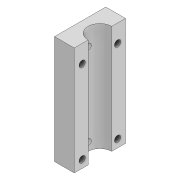
# Autodesk Inventor part: Tube_outerhole_template_p2
Saved by Autodesk Inventor 2022 (Build 260153000, 153)
## iProperties
Created: 2022-05-02
Part Number: Tube_outerhole_template_p2
Material: Generic
Document SubType Name: Modeling
Designer: dell
Density: 1 g/cm^3
Appearance: Default
Author: dell
Autodesk Inventor part; units mm, degrees
ref_plane "YZ Plane" through (0, 0, 0) normal (1, 0, 0) x (0, 1, 0)
ref_plane "XZ Plane" through (0, 0, 0) normal (0, 1, 0) x (-1, 0, 0)
ref_plane "XY Plane" through (0, 0, 0) normal (0, 0, 1) x (1, 0, 0)
sketch "Sketch1" plane through (0, 0, 0) normal (0, 1, 0) x (-1, 0, 0)
  circle A0 centre (0, 0) radius 6
  line L0 (10, 13) -> (-10, 13)
  line L1 (-10, 13) -> (-10, -13)
  line L2 (-10, -13) -> (10, -13)
  line L3 (10, -13) -> (10, 13)
  dimension "d0" = 12
  dimension "d1" = 10
  dimension "d2" = 10
  dimension "d3" = 13
  dimension "d4" = 13
  constraints: 8 end point, 2 parallel, 1 centre point, 1 coincident, 1 horizontal, 1 perpendicular
  measures "d0" diameter of A0
  measures "d1" distance from line of point (0, 0) L1
  measures "d2" distance from line of point (0, 0) L3
  measures "d3" distance from line of point (0, 0) L2
  measures "d4" distance from line of point (0, 0) L0
extrude "Extrusion1" add sketch "Sketch1" along normal blind 55
sketch "Sketch2" plane through (10, 0, 13) normal (1, 0, 0) x (0, 0, -1)
  circle A0 centre (13, 4) radius 1.55
  line L0 (0, 0) -> (26, 0) projected
  circle A1 centre (13, 46) radius 1.55
  line L1 (0, 0) -> (0, 55) projected
  point P0 (13, 0)
  dimension "d7" = 3.1
  dimension "d8" = 4
  dimension "d9" = 3.1
  dimension "d10" = 46
  dimension "d11" = 13
  dimension "d12" = 13
  constraints: 2 centre point
  measures "d7" diameter of A0
  measures "d8" distance from line of L0 A0.centre
  measures "d9" diameter of A1
  measures "d10" distance from line of L0 A1.centre
  measures "d11" distance from line of L1 A0.centre
  measures "d12" distance from line of L1 A1.centre
extrude "Extrusion2" cut sketch "Sketch2" against normal blind 55
sketch "Sketch3" plane through (10, 0, 13) normal (1, 0, 0) x (0, 0, -1)
  circle A0 centre (13, 4) radius 1.55 projected
  circle A1 centre (13, 46) radius 1.55 projected
  line L0 (0, 0) -> (26, 0) projected
  line L1 (26, 0) -> (26, 55) projected
  line L2 (0, 55) -> (26, 55) projected
  line L3 (0, 0) -> (0, 55) projected
  circle A2 centre (13, 46) radius 3.55
  circle A3 centre (13, 4) radius 3.55
  circle A4 centre (4, 46) radius 1.6
  circle A5 centre (22, 46) radius 1.6
  circle A6 centre (4, 4) radius 1.6
  circle A7 centre (22, 4) radius 1.6
  point P0 (13, 0)
  dimension "d15" = 2
  dimension "d16" = 2
  dimension "d19" = 3.2
  dimension "d20" = 3.2
  dimension "d21" = 3.2
  dimension "d22" = 3.2
  dimension "d23" = 4
  dimension "d24" = 4
  dimension "d25" = 4
  dimension "d26" = 4
  constraints: 6 centre point
  measures "d15" radial gap between concentric circles of A1 A2
  measures "d16" radial gap between concentric circles of A0 A3
  measures "d19" diameter of A4
  measures "d20" diameter of A5
  measures "d21" diameter of A6
  measures "d22" diameter of A7
  measures "d23" distance from line of L3 A6.centre
  measures "d24" distance from line of L1 A7.centre
  measures "d25" distance from line of L3 A4.centre
  measures "d26" distance from line of L1 A5.centre
extrude "Extrusion3" add sketch "Sketch3" along normal blind 6 contours A2 | A3
extrude "Extrusion4" cut sketch "Sketch3" against normal blind 100 contours A4 | A5 | A6 | A7
sketch "Sketch5" plane through (0, 0, 0) normal (0, -1, 0) x (1, 0, 0)
  line L0 (0, 24.0189) -> (-16.1408, 24.0189)
  line L1 (-16.1408, 24.0189) -> (-16.1408, -21.0721)
  line L2 (-16.1408, -21.0721) -> (0, -21.0721)
  line L3 (0, -21.0721) -> (0, 24.0189)
  line L4 (-23.7707, -26.6878) -> (26.2299, -26.6878)
  line L5 (26.2299, -26.6878) -> (26.2299, 29.3211)
  line L6 (26.2299, 29.3211) -> (-23.7707, 29.3211)
  line L7 (-23.7707, 29.3211) -> (-23.7707, -26.6878)
  point P0 (0, 0)
  constraints: 16 end point, 4 parallel, 2 horizontal, 2 perpendicular
extrude "Extrusion5" cut sketch "Sketch5" against normal blind 100
body "Solid1"
